Autodesk Inventor part; units mm, degrees
(part 2 of 2)
  spline S120 degree 2 poles (-62.2926, 68.523) (-62.2926, 68.0417) (-62.8268, 67.2285) (-63.7796, 66.8098) (-64.5111, 66.8098) knots 0 0 0 1 2 3 3 3
  spline S121 degree 2 poles (-64.5111, 66.8098) (-65.7863, 66.8098) (-66.7729, 67.7915) (-66.8354, 68.5519) knots 0 0 0 1 2 2 2
  line L170 (-61.7873, 68.5519) -> (-60.3147, 68.6433)
  spline S122 degree 2 poles (-60.3147, 68.6433) (-60.2666, 68.2824) (-60.1222, 68.0947) knots 0 0 0 1 1 1
  spline S123 degree 2 poles (-60.1222, 68.0947) (-59.8816, 67.7915) (-59.4341, 67.7915) knots 0 0 0 1 1 1
  spline S124 degree 2 poles (-59.4341, 67.7915) (-59.1068, 67.7915) (-58.7459, 68.1043) (-58.7459, 68.3064) knots 0 0 0 1 2 2 2
  spline S125 degree 2 poles (-58.7459, 68.3064) (-58.7459, 68.4989) (-58.9192, 68.6529) knots 0 0 0 1 1 1
  spline S126 degree 2 poles (-58.9192, 68.6529) (-59.0876, 68.8069) (-59.7084, 68.9465) knots 0 0 0 1 1 1
  spline S127 degree 2 poles (-59.7084, 68.9465) (-60.7286, 69.1726) (-61.1617, 69.5528) knots 0 0 0 1 1 1
  spline S128 degree 2 poles (-61.1617, 69.5528) (-61.5996, 69.933) (-61.5996, 70.5201) knots 0 0 0 1 1 1
  spline S129 degree 2 poles (-61.5996, 70.5201) (-61.5996, 70.9051) (-61.1521, 71.5884) (-60.2522, 71.983) (-59.4726, 71.983) knots 0 0 0 1 2 3 3 3
  spline S130 degree 2 poles (-59.4726, 71.983) (-58.5101, 71.983) (-57.5043, 71.2708) (-57.4081, 70.4912) knots 0 0 0 1 2 2 2
  line L171 (-57.4081, 70.4912) -> (-58.8662, 70.4046)
  spline S131 degree 2 poles (-58.8662, 70.4046) (-58.924, 70.7415) (-59.2993, 71.0494) (-59.6266, 71.0494) knots 0 0 0 1 2 2 2
  spline S132 degree 2 poles (-59.6266, 71.0494) (-59.8961, 71.0494) (-60.1704, 70.8233) (-60.1704, 70.6548) knots 0 0 0 1 2 2 2
  spline S133 degree 2 poles (-60.1704, 70.6548) (-60.1704, 70.5393) (-60.0549, 70.4431) knots 0 0 0 1 1 1
  spline S134 degree 2 poles (-60.0549, 70.4431) (-59.9442, 70.342) (-59.5351, 70.2602) knots 0 0 0 1 1 1
  spline S135 degree 2 poles (-59.5351, 70.2602) (-58.5197, 70.0389) (-57.6439, 69.5913) (-57.2445, 68.932) (-57.2445, 68.523) knots 0 0 0 1 2 3 3 3
  spline S136 degree 2 poles (-57.2445, 68.523) (-57.2445, 68.0417) (-57.7786, 67.2285) (-58.7315, 66.8098) (-59.4629, 66.8098) knots 0 0 0 1 2 3 3 3
  spline S137 degree 2 poles (-59.4629, 66.8098) (-60.7382, 66.8098) (-61.7247, 67.7915) (-61.7873, 68.5519) knots 0 0 0 1 2 2 2
  point P0 (0, 0)
  point P1 (-8, 83)
  point P2 (8, 83)
  point P3 (-83, 8)
  point P4 (83, 73)
  point P5 (83, 8)
  dimension "d46" = 45
  dimension "d47" = 20
  dimension "d48" = 40
  dimension "d49" = 20
  constraints: 2 horizontal alignment, 2 vertical, 2 vertical alignment, 1 midpoint, 4 other
  measures "d46" distance of L4.start L4.end
  measures "d47" distance of L6.end L4.start
  measures "d48" distance of L0.start L0.end
  measures "d49" distance of L0.end L1.end
extrude "Extrusion3" cut sketch "Sketch3" against normal blind 1
equation "\"d34\" = d33"
body "Solid1"
